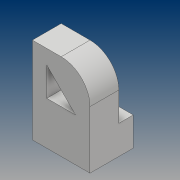
# Autodesk Inventor part: 37(54283.185 mm^3)
Saved by Autodesk Inventor 2018 (Build 220112000, 112)
## iProperties
Created: 2020-09-18
Part Number: 37(54283.185 mm^3)
Material: 一般
Document SubType Name: Modeling
Designer: 88697
Density: 1 g/cm^3
Appearance: 預設
Author: 88697
Autodesk Inventor part; units mm, degrees
ref_plane "YZ Plane" through (0, 0, 0) normal (1, 0, 0) x (0, 1, 0)
ref_plane "XZ Plane" through (0, 0, 0) normal (0, 1, 0) x (-1, 0, 0)
ref_plane "XY Plane" through (0, 0, 0) normal (0, 0, 1) x (1, 0, 0)
sketch "草圖1" plane through (0, 0, 0) normal (0, 1, 0) x (-1, 0, 0)
  line L0 (0, 0) -> (-40, 0)
  line L1 (-40, 0) -> (-40, -60)
  line L2 (-40, -60) -> (0, -60)
  line L3 (0, -60) -> (0, 0)
  dimension "d0" = 40
  dimension "d1" = 60
  constraints: 8 end point, 2 parallel, 1 horizontal, 1 perpendicular
  measures "d0" distance of L0.start L0.end
  measures "d1" distance of L0.end L1.end
extrude "擠出1" add sketch "草圖1" along normal blind 20
sketch "草圖2" plane through (40, 0, -60) normal (0, 0, -1) x (-1, 0, 0)
  line L0 (40, 20) -> (0, 20) projected
  line L1 (40, 20) -> (40, 40)
  line L2 (40, 40) -> (30, 40)
  line L3 (30, 40) -> (10, 30)
  line L4 (10, 30) -> (0, 30)
  line L5 (0, 30) -> (0, 20)
  line L6 (0, 0) -> (40, 0) projected
  dimension "d4" = 40
  dimension "d5" = 10
  dimension "d6" = 10
  dimension "d7" = 10
  constraints: 10 end point, 2 perpendicular, 1 parallel, 1 vertical
  measures "d4" distance between parallel lines of L6 L2
  measures "d5" distance of L1.end L2.end
  measures "d6" distance from line of L3.end L5
  measures "d7" distance between parallel lines of L2 L4
extrude "擠出2" add sketch "草圖2" against normal blind 20
fillet "圓角1" radius 20 1 edges at (40, 10, 0)
sketch "草圖3" plane through (0, 20, 0) normal (0, 1, 0) x (1, 0, 0)
  line L0 (10, 30) -> (30, 30)
  line L1 (30, 30) -> (10, 10)
  line L2 (10, 10) -> (10, 30)
  line L3 (0, 40) -> (0, 0) projected
  line L4 (0, 0) -> (20, 0) projected
  line L5 (30, 40) -> (10, 40) projected
  line L6 (40, 20) -> (40, 40) projected
  dimension "d11" = 10
  dimension "d12" = 10
  dimension "d13" = 10
  dimension "d14" = 10
  constraints: 6 end point, 1 horizontal, 1 perpendicular
  measures "d11" distance between parallel lines of L3 L2
  measures "d12" distance from line of L4 L1.end
  measures "d13" distance between parallel lines of L0 L5
  measures "d14" distance from line of L6 L0.end
extrude "擠出3" cut sketch "草圖3" against normal blind 20
